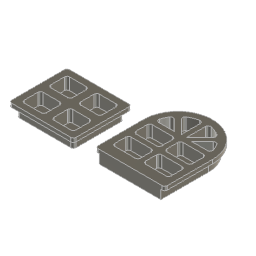
gingerbread-house (Autodesk Fusion 360 design; units mm, degrees)
Autodesk Fusion 360 part; units mm, degrees
sketch "base" plane through (0, 0, 0) normal (0, 0, 1) x (1, 0, 0)
  line L0 (0, 0) -> (22, 0)
  line L1 (22, 0) -> (22, 19.5)
  line L2 (22, 19.5) -> (0, 19.5)
  line L3 (0, 19.5) -> (0, 0)
  line L4 (32, 0) -> (55.8, 0)
  line L5 (55.8, 0) -> (55.8, 18.5)
  line L6 (32, 18.5) -> (32, 0)
  arc A0 (55.8, 18.5) -> (32, 18.5) centre (43.9, 18.5) ccw
  line L7 (32, 18.5) -> (55.8, 18.5) construction
  circle A1 centre (11.9872, 42.3549) radius 9.65
  dimension "d1" = 22
  dimension "d2" = 19.5
  dimension "d20" = 23.8
  dimension "d21" = 18.5
  dimension "d22" = 10
  dimension "d47" = 19.3
  dimension "d57" = 11.9
  constraint horizontal L0
  constraint vertical L1
  constraint horizontal L2
  constraint vertical L3
  constraint coincident L0.start L3.end
  constraint horizontal L4
  constraint vertical L5
  constraint vertical L6
  constraint collinear L0 L4
  constraint perpendicular L5 L7
  measures "d1" distance of L0.start L0.end
  measures "d2" distance of L0.start L2.end
  measures "d20" distance of L4.start L4.end
  measures "d21" distance of L4.start L6.start
  measures "d22" distance of L0.end L4.start
  measures "d47" diameter of A1
  measures "d57" radius of A0
extrude "insert" add sketch "base" along normal blind 3.5 makes body 1 at (7.3333, 13, 0) makes body 2 at (47.8667, 12.3333, 0) makes body 3 at (13.1624, 45.3492, 0)
sketch "upper" plane through (0, 0, 3.5) normal (0, 0, 1) x (-1, 0, 0)
  line L0 (0, -19.5) -> (0, 0) construction
  line L1 (0, 0) -> (-22, 0) construction
  line L2 (-22, 0) -> (-22, -19.5) construction
  line L3 (-22, -19.5) -> (0, -19.5) construction
  line L4 (1.5, 1.5) -> (-23.5, 1.5)
  line L5 (-23.5, 1.5) -> (-23.5, -21)
  line L6 (-23.5, -21) -> (1.5, -21)
  line L7 (1.5, -21) -> (1.5, 1.5)
  arc A0 (-55.8, -18.5) -> (-32, -18.5) centre (-43.9, -18.5) ccw construction
  line L8 (-32, -18.5) -> (-32, 0) construction
  line L9 (-55.8, 0) -> (-55.8, -18.5) construction
  line L10 (-32, 0) -> (-55.8, 0) construction
  line L11 (-57.3, 0) -> (-57.3, -18.5)
  arc A1 (-57.3, -18.5) -> (-30.5, -18.5) centre (-43.9, -18.5) ccw
  line L12 (-30.5, -18.5) -> (-30.5, 0)
  line L13 (-30.5, 0) -> (-57.3, 0)
  circle A2 centre (-11.9872, -42.3549) radius 9.65 construction
  circle A3 centre (-11.9872, -42.3549) radius 11.15
  dimension "d5" = 1.5
  dimension "d25" = 1.5
  dimension "d48" = 1.5
  constraint perpendicular L11 L13
  constraint collinear L10 L13
extrude "main" add sketch "upper" along normal blind 1.5 bodies 1 2 3
sketch "face" plane through (0, 0, 5) normal (0, 0, 1) x (-1, 0, 0)
  line L0 (1.5, -21) -> (1.5, 1.5)
  line L1 (1.5, 1.5) -> (-23.5, 1.5)
  line L2 (-23.5, 1.5) -> (-23.5, -21)
  line L3 (-23.5, -21) -> (1.5, -21)
  line L4 (-11, -21) -> (-11, 1.5) construction
  line L5 (1.5, -9.75) -> (-23.5, -9.75) construction
  line L6 (-1, -18.5) -> (-9.5, -18.5)
  line L7 (-9.5, -18.5) -> (-9.5, -11.25)
  line L8 (-9.5, -11.25) -> (-1, -11.25)
  line L9 (-1, -11.25) -> (-1, -18.5)
  line L10 (0, -19.5) -> (0, 0) construction
  line L11 (-22, -19.5) -> (0, -19.5) construction
  line L12 (-21, -18.5) -> (-12.5, -18.5)
  line L13 (-21, -11.25) -> (-21, -18.5)
  line L14 (-12.5, -18.5) -> (-12.5, -11.25)
  line L15 (-12.5, -11.25) -> (-21, -11.25)
  line L16 (-12.5, -8.25) -> (-21, -8.25)
  line L17 (-1, -8.25) -> (-1, -1)
  line L18 (-9.5, -1) -> (-9.5, -8.25)
  line L19 (-12.5, -1) -> (-12.5, -8.25)
  line L20 (-21, -1) -> (-12.5, -1)
  line L21 (-1, -1) -> (-9.5, -1)
  line L22 (-9.5, -8.25) -> (-1, -8.25)
  line L23 (-21, -8.25) -> (-21, -1)
  line L24 (-32, 0) -> (-55.8, 0)
  arc A0 (-55.8, -18.5) -> (-32, -18.5) centre (-43.9, -18.5) ccw
  line L25 (-32, -18.5) -> (-32, 0)
  line L26 (-55.8, 0) -> (-55.8, -18.5)
  arc A1 (-54.8, -18.5) -> (-33, -18.5) centre (-43.9, -18.5) ccw
  line L27 (-54.8, -18.5) -> (-54.8, -4)
  line L28 (-54.8, -4) -> (-33, -4)
  line L29 (-33, -4) -> (-33, -18.5)
  line L30 (-33, -11.25) -> (-54.8, -11.25) construction
  line L31 (-43.9, -4) -> (-43.9, -29.4) construction
  line L32 (-33, -18.5) -> (-54.8, -18.5) construction
  line L33 (-43.9, -18.5) -> (-51.6075, -26.2075) construction
  line L34 (-43.9, -18.5) -> (-33, -18.5) construction
  line L35 (-43.9, -18.5) -> (-36.1925, -26.2075) construction
  line L36 (-43.9, -18.5) -> (-33, -18.5) construction
  line L37 (-44.9, -20.9142) -> (-50.8679, -26.8821)
  line L38 (-42.9, -20.9142) -> (-36.9321, -26.8821)
  line L39 (-33, -10.25) -> (-54.8, -10.25)
  line L40 (-33, -12.25) -> (-54.8, -12.25)
  line L41 (-33, -18.5) -> (-54.8, -18.5)
  line L42 (-42.9, -4) -> (-42.9, -18.5)
  line L43 (-42.9, -20.9142) -> (-42.9, -29.354)
  line L44 (-44.9, -4) -> (-44.9, -19.5)
  line L45 (-44.9, -20.9142) -> (-44.9, -29.354)
  line L46 (-33.1851, -20.5) -> (-40.4858, -20.5)
  line L47 (-47.3142, -20.5) -> (-54.6149, -20.5)
  line L48 (-40.4858, -20.5) -> (-35.5179, -25.4679)
  line L49 (-47.3142, -20.5) -> (-52.2821, -25.4679)
  circle A2 centre (-11.9872, -42.3549) radius 9.65 construction
  line L50 (-20.637, -42.3549) -> (-3.3372, -42.3549) construction
  line L51 (-11.9872, -33.7049) -> (-11.9872, -51.0049) construction
  line L52 (-20.5855, -43.3549) -> (-12.9872, -43.3549)
  line L53 (-10.9872, -43.3549) -> (-3.3952, -43.3549)
  line L54 (-20.5792, -41.3549) -> (-12.9872, -41.3549)
  line L55 (-10.9872, -41.3549) -> (-3.3952, -41.3549)
  line L56 (-12.9872, -33.7629) -> (-12.9872, -41.3549)
  line L57 (-12.9872, -43.3549) -> (-12.9872, -50.9469)
  line L58 (-10.9872, -33.7629) -> (-10.9872, -41.3549)
  line L59 (-10.9872, -43.3549) -> (-10.9872, -50.9469)
  circle A3 centre (-11.9872, -42.3549) radius 11.15
  circle A4 centre (-11.9872, -42.3549) radius 8.65
  dimension "d8" = 1
  dimension "d9" = 1
  dimension "d10" = 3
  dimension "d11" = 3
  dimension "d28" = 135
  dimension "d29" = 45
  dimension "d34" = 1
  dimension "d36" = 1
  dimension "d37" = -1
  dimension "d40" = 4
  dimension "d41" = 1
  dimension "d42" = 1
  dimension "d53" = 1.5
  dimension "d54" = -1
  constraint midpoint L3 L4.start
  constraint midpoint L1 L4.end
  constraint midpoint L0 L5.start
  constraint midpoint L2 L5.end
  constraint horizontal L6
  constraint vertical L7
  constraint horizontal L8
  constraint vertical L9
  constraint symmetric L4 L6.start L12.start
  constraint symmetric L4 L6.end L12.end
  constraint symmetric L4 L7.end L14.end
  constraint symmetric L4 L8.end L13.start
  constraint symmetric L5 L6.start L17.end
  constraint symmetric L5 L6.end L18.start
  constraint symmetric L5 L7.end L18.end
  constraint symmetric L5 L8.end L17.start
  constraint symmetric L5 L12.start L20.start
  constraint symmetric L5 L12.end L19.start
  constraint symmetric L5 L13.start L16.end
  constraint symmetric L5 L14.end L16.start
  constraint coincident A0.centre A1.centre
  constraint tangent A1 L27
  constraint vertical L27
  constraint perpendicular L27 L28
  constraint vertical L29
  constraint midpoint L29 L30.start
  constraint midpoint L27 L30.end
  constraint midpoint L28 L31.start
  constraint midpoint A1 L31.end
  constraint perpendicular L28 L31
  constraint horizontal L34
  constraint horizontal L36
  constraint coincident A1 L38.end
  constraint coincident A1 L48.end
  constraint coincident A1 L35.end
  constraint coincident A1 L33.end
  constraint coincident A1 L37.end
  constraint coincident A1 L49.end
  constraint coincident A1 L47.end
  constraint coincident A1 L46.start
  constraint coincident L29 L40.start
  constraint coincident L29 L39.start
  constraint coincident L27 L40.end
  constraint coincident L27 L39.end
  constraint coincident A1 L29.end
  constraint coincident A1 L43.end
  constraint coincident A1 L45.end
  constraint collinear L42 L43
  constraint coincident L37.start L44
  constraint coincident L33 L44.end
  constraint collinear L44 L45
  constraint collinear L46 L47
  constraint coincident L32 L42.end
  constraint coincident L28 L42.start
  constraint coincident L28 L44.start
  constraint horizontal L50
  constraint perpendicular L50 L51
  constraint coincident A2.centre L50
  constraint coincident A2.centre L51
  constraint coincident L52.end L56
  constraint collinear L52 L53
  constraint coincident L53.start L58
  constraint collinear L54 L55
  constraint collinear L56 L57
  constraint collinear L58 L59
  constraint coincident L51.start A4
  constraint coincident L51.end A4
  constraint coincident L54.start A4
  constraint coincident L53.end A4
  constraint coincident L50.end A4
  constraint coincident L55.end A4
  constraint coincident L57.end A4
  constraint coincident L59.end A4
  constraint coincident L56.start A4
  constraint coincident L58.start A4
  measures "d8" distance of L6 L11
  measures "d9" distance of L9 L10
  measures "d10" distance of L6.end L12.end
  measures "d11" distance of L8.end L17.start
  measures "d28" angle of L33 L34
  measures "d29" angle of L35 L36
  measures "d34" distance of L25 L29
  measures "d40" distance of L24 L28
  measures "d41" distance of L35 L48
  measures "d42" distance of L33 L49
extrude "panes" cut sketch "face" against normal up to surface (4.6 mm away) contours L6 L7 L8 L9 | L12 L13 L14 L15 | L16 L19 L20 L23 | L17 L18 L21 L22 | L27 L40 L41 L44 | A1 L47 L49 | L27 L28 L39 L44 | L29 L40 L41 L42 | A1 L37 L45 | L28 L29 L39 L42 | A1 L46 L48 | A1 L38 L43 | L52 L57 A4 | L54 L56 A4 | L53 L59 A4 | L55 L58 A4 bodies 1 2 3
fillet "Fillet1" radius 1 4 edges at (23.5, -1.5, 4.25) (23.5, 21, 4.25) (-1.5, 21, 4.25) (-1.5, -1.5, 4.25) on bodies 1 2
fillet "Fillet1" radius 1 2 edges at (30.5, 0, 4.25) (57.3, 0, 4.25) on bodies 1 2
fillet "Fillet3" radius 1 4 edges at (22, 19.5, 1.75) (22, 0, 1.75) (0, 19.5, 1.75) (0, 0, 1.75) on bodies 1
fillet "Fillet2" radius 1 28 edges at (21, 1, 2.7) (12.5, 1, 2.7) (9.5, 1, 2.7) (1, 1, 2.7) (1, 8.25, 2.7) (9.5, 8.25, 2.7) (12.5, 8.25, 2.7) (21, 8.25, 2.7) (21, 11.25, 2.7) (12.5, 11.25, 2.7) (21, 18.5, 2.7) (12.5, 18.5, 2.7) (9.5, 18.5, 2.7) (1, 18.5, 2.7) (1, 11.25, 2.7) (9.5, 11.25, 2.7) (3.3952, 43.3549, 2.7) (10.9872, 50.9469, 2.7) (12.9872, 50.9469, 2.7) (20.5792, 43.3549, 2.7) (20.5792, 41.3549, 2.7) (12.9872, 33.7629, 2.7) (10.9872, 33.7629, 2.7) (3.3952, 41.3549, 2.7) (10.9872, 41.3549, 2.7) (10.9872, 43.3549, 2.7) (12.9872, 43.3549, 2.7) (12.9872, 41.3549, 2.7) on bodies 1 2 3
fillet "Fillet2" radius 1 24 edges at (35.5179, 25.4679, 2.7) (33.1851, 20.5, 2.7) (36.9321, 26.8821, 2.7) (42.9, 29.354, 2.7) (44.9, 29.354, 2.7) (50.8679, 26.8821, 2.7) (52.2821, 25.4679, 2.7) (54.6149, 20.5, 2.7) (33, 18.5, 2.7) (33, 12.25, 2.7) (33, 10.25, 2.7) (33, 4, 2.7) (42.9, 10.25, 2.7) (42.9, 4, 2.7) (42.9, 18.5, 2.7) (42.9, 12.25, 2.7) (44.9, 18.5, 2.7) (44.9, 12.25, 2.7) (44.9, 10.25, 2.7) (44.9, 4, 2.7) (54.8, 4, 2.7) (54.8, 10.25, 2.7) (54.8, 12.25, 2.7) (54.8, 18.5, 2.7) on bodies 1 2 3
hidden bodies 3
equation "d37 = -d36"
named bodies: "window-rect", "door", "window-round"
